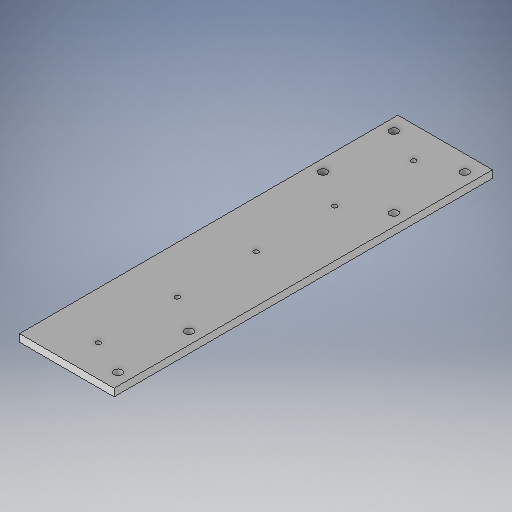
# Autodesk Inventor part: GOES_Mount
Saved by Autodesk Inventor 2025.3 (Build 293356000, 356)
## iProperties
Created: 2025-12-10
Part Number: GOES_Mount
Material: Generic
Document SubType Name: Modeling
Designer: sonata
Density: 1 g/cm^3
Appearance: Default
Author: sonata
Autodesk Inventor part; units mm, degrees
ref_plane "YZ Plane" through (0, 0, 0) normal (1, 0, 0) x (0, 1, 0)
ref_plane "XZ Plane" through (0, 0, 0) normal (0, 1, 0) x (-1, 0, 0)
ref_plane "XY Plane" through (0, 0, 0) normal (0, 0, 1) x (1, 0, 0)
sketch "Sketch1" plane through (0, 0, 0) normal (0, 1, 0) x (-1, 0, 0)
  line L0 (0, 0) -> (76.2, 0)
  line L1 (76.2, 0) -> (76.2, -304.8)
  line L2 (76.2, -304.8) -> (0, -304.8)
  line L3 (0, -304.8) -> (0, 0)
  dimension "d0" = 304.8
  dimension "d1" = 76.2
  constraints: 8 end point, 2 parallel, 1 horizontal, 1 perpendicular
  measures "d0" distance of L0.end L1.end
  measures "d1" distance of L1.end L2.end
extrude "Extrusion1" add sketch "Sketch1" along normal blind 5.9995
sketch "Sketch2" plane through (0, 5.9995, 0) normal (0, 1, 0) x (1, 0, 0)
  line L0 (0, 0) -> (0, 304.8) projected
  line L1 (-76.2, 0) -> (0, 0) projected
  point P0 (-9.525, 12.7)
  point P1 (-9.525, 69.85)
  dimension "d4" = 57.15
  dimension "d5" = 9.525
  dimension "d13" = 12.7
  constraints: 1 vertical alignment
  measures "d4" distance of point (-9.525, 69.85) point (-9.525, 12.7)
  measures "d5" distance from line of point (-9.525, 12.7) L0
  measures "d13" distance from line of point (-9.525, 12.7) L1
hole "Hole1" at (-9.525, 5.9995, -12.7) at (-9.525, 5.9995, -69.85) direction (0, -1, 0) diameter 6.604 end through all
sketch "Sketch3" plane through (0, 5.9995, 0) normal (0, 1, 0) x (1, 0, 0)
  line L0 (0, 0) -> (0, 304.8) projected
  line L1 (-76.2, 304.8) -> (-76.2, 0) projected
  line L2 (0, 304.8) -> (-76.2, 304.8) projected
  point P0 (-9.525, 292.1)
  point P1 (-9.525, 234.95)
  point P2 (-66.675, 234.95)
  point P3 (-66.675, 292.1)
  dimension "d14" = 57.15
  dimension "d15" = 9.525
  dimension "d16" = 9.525
  dimension "d17" = 12.7
  constraints: 2 horizontal alignment, 2 vertical alignment
  measures "d14" distance of point (-66.675, 292.1) point (-66.675, 234.95)
  measures "d15" distance from line of L0 point (-9.525, 292.1)
  measures "d16" distance from line of L1 point (-66.675, 292.1)
  measures "d17" distance from line of L2 point (-66.675, 292.1)
hole "Hole2" at (-9.525, 5.9995, -292.1) at (-9.525, 5.9995, -234.95) at (-66.675, 5.9995, -234.95) at (-66.675, 5.9995, -292.1) direction (0, -1, 0) diameter 6.604 end through all
sketch "Sketch4" plane through (0, 0, 0) normal (0, -1, 0) x (1, 0, 0)
  line L0 (0, -304.8) -> (-76.2, -304.8) projected
  line L1 (-76.2, 0) -> (0, 0) projected
  line L2 (-76.2, -304.8) -> (-76.2, 0) projected
  point P0 (-38.1, -279.4)
  point P1 (-38.1, -215.9)
  point P2 (-38.1, -152.4)
  point P3 (-38.1, -88.9)
  point P4 (-38.1, -25.4)
  dimension "d25" = 25.4
  dimension "d26" = 25.4
  dimension "d27" = 63.5
  dimension "d28" = 63.5
  dimension "d29" = 63.5
  dimension "d30" = 38.1
  constraints: 4 vertical alignment
  measures "d25" distance from line of L0 point (-38.1, -279.4)
  measures "d26" distance from line of L1 point (-38.1, -25.4)
  measures "d27" distance of point (-38.1, -215.9) point (-38.1, -279.4)
  measures "d28" distance of point (-38.1, -152.4) point (-38.1, -215.9)
  measures "d29" distance of point (-38.1, -88.9) point (-38.1, -152.4)
  measures "d30" distance from line of L2 point (-38.1, -279.4)
hole "Hole3" at (-38.1, 0, -279.4) at (-38.1, 0, -215.9) at (-38.1, 0, -152.4) at (-38.1, 0, -88.9) at (-38.1, 0, -25.4) direction (0, 1, 0) diameter 3.81 end through all clearance for "Flat Head Machine Screw (82)" size "#6" standard "Ansi Unified Screw Threads"
body "Solid1"
